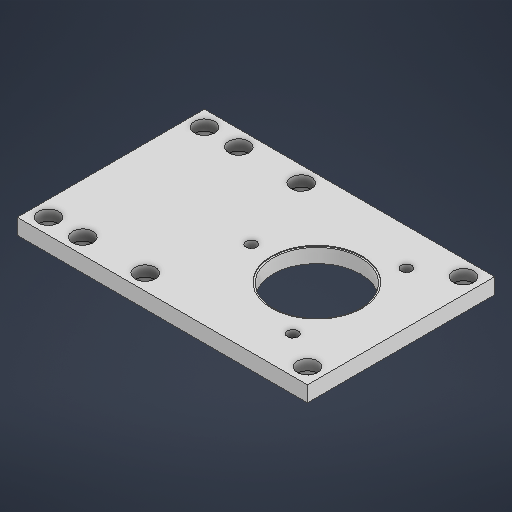
# Autodesk Inventor part: plate 2
Saved by Autodesk Inventor 2025.2 (Build 292293000, 293)
## iProperties
Created: 2025-04-19
Part Number: plate 2
Material: Generic
Document SubType Name: Modeling
Designer: klawy
Density: 1 g/cm^3
Appearance: Default
Author: klawy
Autodesk Inventor part; units mm, degrees
ref_plane "YZ Plane" through (0, 0, 0) normal (1, 0, 0) x (0, 1, 0)
ref_plane "XZ Plane" through (0, 0, 0) normal (0, 1, 0) x (-1, 0, 0)
ref_plane "XY Plane" through (0, 0, 0) normal (0, 0, 1) x (1, 0, 0)
sketch "Sketch1" plane through (0, 0, 0) normal (0, 1, 0) x (-1, 0, 0)
  line L0 (46.5, 30) -> (-46.5, 30)
  line L1 (-46.5, 30) -> (-46.5, -30)
  line L2 (-46.5, -30) -> (46.5, -30)
  line L3 (46.5, -30) -> (46.5, 30)
  line L4 (46.5, 30) -> (-46.5, -30) construction
  line L5 (-46.5, 30) -> (46.5, -30) construction
  circle A0 centre (-19.5, 0) radius 12.5
  line L6 (152.1746, 0) -> (-152.1746, 0) construction
  line L7 (0, 58.0523) -> (0, -58.0523) construction
  point P0 (0, 0)
  dimension "d0" = 93
  dimension "d2" = 25
  dimension "d4" = 60
  dimension "d5" = 27
  constraints: 16 end point, 4 midpoint, 2 horizontal, 2 parallel, 1 centre point, 1 perpendicular, 1 point on line, 1 vertical
  measures "d0" distance of L1.end L2.end
  measures "d2" diameter of A0
  measures "d4" distance of L0.end L1.end
  measures "d5" distance from line of L1 A0.centre
extrude "Extrusion1" add sketch "Sketch1" along normal blind 5
sketch "Sketch2" plane through (0, 5, 0) normal (0, 1, 0) x (1, 0, 0)
  line L0 (-41.5, -25) -> (41.5, -25) construction
  line L1 (41.5, -25) -> (41.5, 25) construction
  line L2 (41.5, 25) -> (-41.5, 25) construction
  line L3 (-41.5, 25) -> (-41.5, -25) construction
  line L4 (-41.5, -25) -> (41.5, 25) construction
  line L5 (41.5, -25) -> (-41.5, 25) construction
  line L6 (46.5, 30) -> (-46.5, 30) projected
  line L7 (46.5, -30) -> (46.5, 30) projected
  point P0 (0, 0)
  dimension "d11" = 5
  dimension "d12" = 5
  constraints: 12 end point, 4 coincident, 2 midpoint, 2 parallel, 1 horizontal, 1 perpendicular
  measures "d11" distance between parallel lines of L6 L2
  measures "d12" distance between parallel lines of L7 L1
hole "Hole1" at (-41.5, 5, -25) at (41.5, 5, -25) at (41.5, 5, 25) at (-41.5, 5, 25) direction (0, -1, 0) diameter 3.4 end through all counterbore diameter 6.5 counterbore depth 3.4 clearance for "Socket Head Cap Screw ISO 4762" size "M3" standard "ISO"
sketch "Sketch3" plane through (0, 0, 0) normal (0, -1, 0) x (1, 0, 0)
  circle A0 centre (-41.5, 25) radius 3.25 projected
  circle A1 centre (-41.5, 25) radius 4
  circle A2 centre (-41.5, 25) radius 1.7 projected
  circle A3 centre (41.5, 25) radius 1.7 projected
  circle A4 centre (41.5, -25) radius 1.7 projected
  circle A5 centre (-41.5, -25) radius 1.7 projected
  line L0 (46.5, 30) -> (46.5, -30) projected
  line L1 (-46.5, 30) -> (46.5, 30) projected
  line L2 (-46.5, -30) -> (-46.5, 30) projected
  line L3 (46.5, -30) -> (-46.5, -30) projected
  circle A6 centre (41.5, 25) radius 4
  circle A7 centre (-41.5, -25) radius 4
  circle A8 centre (41.5, -25) radius 4
  point P0 (0, 0)
  dimension "d22" = 83
  dimension "d25" = 50
  dimension "d28" = 8
  constraints: 4 centre point, 1 coincident, 1 horizontal, 1 vertical, 6 other
  measures "d22" distance of A1.centre A6.centre
  measures "d25" distance of A1.centre A7.centre
  measures "d28" diameter of A1
extrude "Extrusion2" cut sketch "Sketch3" against normal blind 1 contours A0 | A1 | A2 | A3 | A4 | A5 | A6 | A7 | A8
sketch "Sketch4" plane through (0, 0, 0) normal (0, -1, 0) x (1, 0, 0)
  circle A0 centre (41.5, -25) radius 4 projected
  circle A1 centre (-41.5, -25) radius 4 projected
  circle A2 centre (41.5, 25) radius 4 projected
  circle A3 centre (-41.5, 25) radius 4 projected
  line L0 (46.5, 30) -> (46.5, -30) projected
  line L1 (-46.5, 30) -> (46.5, 30) projected
  line L2 (-46.5, -30) -> (-46.5, 30) projected
  line L3 (46.5, -30) -> (-46.5, -30) projected
  circle A4 centre (19.5, 0) radius 12.5 projected
  circle A5 centre (19.5, 0) radius 14
  point P0 (0, 0)
  dimension "d31" = 28
  constraints: 1 centre point, 1 coincident
  measures "d31" diameter of A5
extrude "Extrusion3" cut sketch "Sketch4" against normal through all contours A5
sketch "Sketch5" plane through (0, 0, 0) normal (0, -1, 0) x (1, 0, 0)
  line L0 (-35.5, 30) -> (-5.5, 30) construction
  line L1 (-5.5, 30) -> (-5.5, -30) construction
  line L2 (-5.5, -30) -> (-35.5, -30) construction
  line L3 (-35.5, -30) -> (-35.5, 30) construction
  line L4 (-65.1, 0) -> (65.1, 0) projected
  circle A0 centre (-30.5, 25) radius 4
  circle A1 centre (-10.5, 25) radius 4
  circle A2 centre (-30.5, -25) radius 4
  circle A3 centre (-10.5, -25) radius 4
  line L5 (-35.5, 30) -> (-5.5, -30) construction
  line L6 (-46.5, -30) -> (-46.5, 30) projected
  point P0 (0, 0)
  point P1 (-35.5, 0)
  point P2 (-20.5, 0)
  dimension "d34" = 60
  dimension "d35" = 30
  dimension "d36" = 8
  dimension "d37" = 5
  dimension "d38" = 5
  dimension "d41" = 20
  dimension "d44" = 50
  dimension "d47" = 26
  constraints: 10 end point, 4 centre point, 2 horizontal, 2 midpoint, 2 parallel, 1 perpendicular, 1 point on line, 1 vertical, 6 other
  measures "d34" distance of L2.end L0.start
  measures "d35" distance of L0.start L0.end
  measures "d36" diameter of A0
  measures "d37" distance from line of L0 A0.centre
  measures "d38" distance from line of L3 A0.centre
  measures "d41" distance of A0.centre A1.centre
  measures "d44" distance of A0.centre A2.centre
  measures "d47" distance from line of L6 point (-20.5, 0)
extrude "Extrusion4" cut sketch "Sketch5" against normal blind 1
sketch "Sketch7" plane through (0, 5, 0) normal (0, 1, 0) x (1, 0, 0)
  circle A0 centre (-30.5, -25) radius 4 construction
  point P0 (0, 0)
  constraints: 1 coincident
hole "Hole2" at (-30.5, 5, 25) direction (0, -1, 0) diameter 3.4 end through all counterbore diameter 6.5 counterbore depth 3.4 clearance for "Socket Head Cap Screw ISO 4762" size "M3" standard "ISO"
pattern_linear "Rectangular Pattern1" count 2 spacing 50 along (0, 0, -1) count 2 spacing 20 along (1, 0, 0) of "Hole2"
sketch "Sketch8" plane through (0, 5, 0) normal (0, 1, 0) x (1, 0, 0)
  circle A0 centre (19.5, 0) radius 12.5 projected
  circle A1 centre (19.5, 0) radius 21 construction
  line L0 (65.1, 0) -> (-65.1, 0) projected
  point P0 (0, 0)
  point P1 (-1.5, 0)
  point P2 (30, -18.1865)
  point P3 (30, 18.1865)
  dimension "d63" = 42
  dimension "d66" = 360
  constraints: 1 coincident, 1 horizontal alignment, 1 point on line, 6 other
hole "Hole3" at (-1.5, 5, 0) at (30, 5, 18.1865) at (30, 5, -18.1865) direction (0, -1, 0) diameter 3.4 end through all clearance for "Socket Head Cap Screw ISO 4762" size "M3" standard "ISO"
sketch "Sketch11" plane through (0, 0, 0) normal (0, -1, 0) x (1, 0, 0)
  circle A0 centre (19.5, 0) radius 14 projected
  circle A1 centre (19.5, 0) radius 14.5
  circle A2 centre (19.5, 0) radius 14 projected
  point P0 (0, 0)
  dimension "d81" = 0.5
  constraints: 1 centre point, 1 coincident
  measures "d81" radial gap between concentric circles of A1 A0
extrude "Extrusion6" cut sketch "Sketch11" against normal blind 0.25
sketch "Sketch12" plane through (0, 5, 0) normal (0, 1, 0) x (1, 0, 0)
  circle A0 centre (19.5, 0) radius 14 projected
  circle A1 centre (19.5, 0) radius 14.5
  point P0 (0, 0)
  dimension "d84" = 0.5
  constraints: 1 centre point, 1 coincident
  measures "d84" radial gap between concentric circles of A0 A1
extrude "Extrusion7" cut sketch "Sketch12" against normal blind 0.25
body "Solid1"
